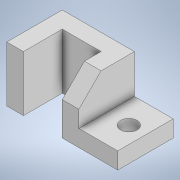
# Autodesk Inventor part: ch2-adjuster
Saved by Autodesk Inventor 2020 (Build 240168000, 168)
## iProperties
Created: 2020-01-24
Part Number: ch2-adjuster
Material: Generic
Document SubType Name: Modeling
Designer: Eric
Density: 1 g/cm^3
Appearance: Default
Author: Eric
Autodesk Inventor part; units mm, degrees
ref_plane "YZ Plane" through (0, 0, 0) normal (1, 0, 0) x (0, 1, 0)
ref_plane "XZ Plane" through (0, 0, 0) normal (0, 1, 0) x (-1, 0, 0)
ref_plane "XY Plane" through (0, 0, 0) normal (0, 0, 1) x (1, 0, 0)
sketch "baseSketch" plane through (0, 0, 0) normal (0, 0, 1) x (1, 0, 0)
  line L0 (0, 63.5) -> (0, 0)
  line L1 (0, 0) -> (63.5, 0)
  line L2 (63.5, 0) -> (63.5, 19.05)
  line L3 (63.5, 19.05) -> (19.05, 19.05)
  line L4 (19.05, 19.05) -> (19.05, 63.5)
  line L5 (19.05, 63.5) -> (0, 63.5)
  dimension "d0" = 63.5
  dimension "d1" = 63.5
  dimension "d2" = 19.05
  dimension "d3" = 19.05
  constraints: 12 end point, 5 perpendicular, 1 coincident, 1 vertical
  measures "d0" distance of L0.start L0.end
  measures "d1" distance of L0.end L1.end
  measures "d2" distance of L1.end L2.end
  measures "d3" distance of L4.end L0.start
extrude "baseExtrude" add sketch "baseSketch" along normal blind 63.5
sketch "Sketch2" plane through (0, 63.5, 0) normal (0, 1, 0) x (1, 0, 0)
  line L0 (0, 0) -> (-63.5, 0)
  line L1 (-63.5, 0) -> (-63.5, -63.5)
  line L2 (-63.5, -63.5) -> (-44.45, -63.5)
  line L3 (-44.45, -63.5) -> (-44.45, -19.05)
  line L4 (-44.45, -19.05) -> (0, -19.05)
  line L5 (0, -19.05) -> (0, 0)
  point P0 (0, 0)
  dimension "d6" = 63.5
  dimension "d7" = 63.5
  dimension "d8" = 19.05
  dimension "d9" = 19.05
  constraints: 12 end point, 5 perpendicular, 1 coincident, 1 horizontal
  measures "d6" distance of L0.end L1.end
  measures "d7" distance of L0.start L0.end
  measures "d8" distance of L4.end L0.start
  measures "d9" distance of L1.end L2.end
extrude "Extrusion2" add sketch "Sketch2" against normal blind 63.5
sketch "Sketch3" plane through (19.05, 19.05, 0) normal (0, 1, 0) x (1, 0, 0)
  circle A0 centre (25.4, -31.75) radius 9.525
  line L0 (44.45, 0) -> (44.45, -63.5) projected
  line L1 (44.45, 0) -> (0, 0) projected
  point P0 (-19.05, 0)
  dimension "d12" = 19.05
  dimension "d13" = 19.05
  dimension "d14" = 31.75
  constraints: 1 centre point
  measures "d12" diameter of A0
  measures "d13" distance from line of L0 A0.centre
  measures "d14" distance from line of L1 A0.centre
extrude "Extrusion3" cut sketch "Sketch3" against normal through all
sketch "Sketch4" plane through (19.05, 19.05, 0) normal (1, 0, 0) x (0, 0, -1)
  line L0 (-63.5, 44.45) -> (-19.05, 44.45) projected
  line L1 (-38.1, 44.45) -> (-63.5, 19.05)
  line L2 (-63.5, 44.45) -> (-63.5, -19.05) projected
  line L3 (-63.5, 19.05) -> (-63.5, 44.45)
  line L4 (-63.5, 44.45) -> (-38.1, 44.45)
  point P0 (0, -19.05)
  dimension "d17" = 25.4
  dimension "d18" = 45
  constraints: 6 end point, 2 point on line, 1 perpendicular, 1 vertical
  measures "d17" distance of L1.start L0.start
  measures "d18" angle of L0 L1
extrude "Extrusion4" cut sketch "Sketch4" against normal up to surface (19.05 mm away)
body "Solid1"
